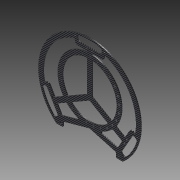
# Autodesk Inventor part: Bottom Plate
Saved by Autodesk Inventor 2015 (Build 190159000, 159)
## iProperties
Created: 2016-08-08
Part Number: Bottom Plate
Material: Generic
Document SubType Name: Modeling
Designer: James Yelland
Density: 1 g/cm^3
Appearance: Default
Mass: 31.8774 g
Surface Area: 332.808 cm^2
Volume: 31.8774 cm^3
Author: James Yelland
Autodesk Inventor part; units mm, degrees
ref_plane "YZ Plane" through (0, 0, 0) normal (1, 0, 0) x (0, 1, 0)
ref_plane "XZ Plane" through (0, 0, 0) normal (0, 1, 0) x (-1, 0, 0)
ref_plane "XY Plane" through (0, 0, 0) normal (0, 0, 1) x (1, 0, 0)
sketch "Sketch1" plane through (0, 0, 0) normal (0, 1, 0) x (-1, 0, 0)
  line L0 (-76.2102, -44) -> (-65.7102, -62.1865)
  line L1 (-67.1743, -67.6506) -> (-69.6351, -69.0713)
  line L2 (-94.6351, -25.7701) -> (-92.1743, -24.3494)
  line L3 (-86.7102, -25.8135) -> (-76.2102, -44)
  arc A0 (-96.4496, -30.438) -> (-74.5849, -68.3088) centre (0, 0) ccw
  arc A1 (-94.6351, -25.7701) -> (-96.4496, -30.438) centre (-92.6351, -29.2342) ccw
  arc A2 (-86.7102, -25.8135) -> (-92.1743, -24.3494) centre (-90.1743, -27.8135) ccw
  arc A3 (-67.1743, -67.6506) -> (-65.7102, -62.1865) centre (-69.1743, -64.1865) ccw
  arc A4 (-74.5849, -68.3088) -> (-69.6351, -69.0713) centre (-71.6351, -65.6072) ccw
  line L4 (76.2102, -44) -> (86.7102, -25.8135)
  line L5 (92.1743, -24.3494) -> (94.6351, -25.7701)
  line L6 (69.6351, -69.0713) -> (67.1743, -67.6506)
  line L7 (65.7102, -62.1865) -> (76.2102, -44)
  arc A5 (74.5849, -68.3088) -> (96.4496, -30.438) centre (0, 0) ccw
  arc A6 (69.6351, -69.0713) -> (74.5849, -68.3088) centre (71.6351, -65.6072) ccw
  arc A7 (65.7102, -62.1865) -> (67.1743, -67.6506) centre (69.1743, -64.1865) ccw
  arc A8 (92.1743, -24.3494) -> (86.7102, -25.8135) centre (90.1743, -27.8135) ccw
  arc A9 (96.4496, -30.438) -> (94.6351, -25.7701) centre (92.6351, -29.2342) ccw
  line L8 (0, 88) -> (-21, 88)
  line L9 (-25, 92) -> (-25, 94.8414)
  line L10 (25, 94.8414) -> (25, 92)
  line L11 (21, 88) -> (0, 88)
  arc A10 (21.8647, 98.7468) -> (-21.8647, 98.7468) centre (0, 0) ccw
  arc A11 (25, 94.8414) -> (21.8647, 98.7468) centre (21, 94.8414) ccw
  arc A12 (21, 88) -> (25, 92) centre (21, 92) ccw
  arc A13 (-25, 92) -> (-21, 88) centre (-21, 92) ccw
  arc A14 (-21.8647, 98.7468) -> (-25, 94.8414) centre (-21, 94.8414) ccw
  line L12 (-75.1122, -39.9019) -> (-77.6122, -35.5718)
  line L13 (-77.6122, -35.5718) -> (-75.8801, -34.5718)
  line L14 (-75.8801, -34.5718) -> (-73.3801, -38.9019)
  line L15 (-73.3801, -38.9019) -> (-75.1122, -39.9019)
  line L16 (-72.1122, -45.0981) -> (-69.6122, -49.4282)
  line L17 (-69.6122, -49.4282) -> (-67.8801, -48.4282)
  line L18 (-67.8801, -48.4282) -> (-70.3801, -44.0981)
  line L19 (-70.3801, -44.0981) -> (-72.1122, -45.0981)
  line L20 (72.1122, -45.0981) -> (69.6122, -49.4282)
  line L21 (69.6122, -49.4282) -> (67.8801, -48.4282)
  line L22 (67.8801, -48.4282) -> (70.3801, -44.0981)
  line L23 (70.3801, -44.0981) -> (72.1122, -45.0981)
  line L24 (73.3801, -38.9019) -> (75.1122, -39.9019)
  line L25 (75.8801, -34.5718) -> (73.3801, -38.9019)
  line L26 (77.6122, -35.5718) -> (75.8801, -34.5718)
  line L27 (75.1122, -39.9019) -> (77.6122, -35.5718)
  line L28 (3, 85) -> (8, 85)
  line L29 (8, 85) -> (8, 83)
  line L30 (8, 83) -> (3, 83)
  line L31 (3, 83) -> (3, 85)
  line L32 (-3, 83) -> (-3, 85)
  line L33 (-8, 83) -> (-3, 83)
  line L34 (-8, 85) -> (-8, 83)
  line L35 (-3, 85) -> (-8, 85)
  line L36 (0, 73.3) -> (-1.5, 73.3)
  line L37 (0, 73.3) -> (1.5, 73.3)
  line L38 (1.5, 73.3) -> (1.5, 74.8)
  line L39 (1.5, 74.8) -> (-1.5, 74.8)
  line L40 (-1.5, 74.8) -> (-1.5, 73.3)
  line L41 (0, 72.7) -> (-1.5, 72.7)
  line L42 (-1.5, 72.7) -> (-1.5, 71.2)
  line L43 (-1.5, 71.2) -> (1.5, 71.2)
  line L44 (1.5, 71.2) -> (1.5, 72.7)
  line L45 (1.5, 72.7) -> (0, 72.7)
  line L46 (-15.0457, 71.3993) -> (-16.5457, 71.3993)
  line L47 (-15.0457, 71.3993) -> (-13.5457, 71.3993)
  line L48 (-13.5457, 71.3993) -> (-13.5457, 72.8993)
  line L49 (-13.5457, 72.8993) -> (-16.5457, 72.8993)
  line L50 (-16.5457, 72.8993) -> (-16.5457, 71.3993)
  line L51 (-15.0457, 70.7993) -> (-16.5457, 70.7993)
  line L52 (-16.5457, 70.7993) -> (-16.5457, 69.2993)
  line L53 (-16.5457, 69.2993) -> (-13.5457, 69.2993)
  line L54 (-13.5457, 69.2993) -> (-13.5457, 70.7993)
  line L55 (-13.5457, 70.7993) -> (-15.0457, 70.7993)
  line L56 (-29.1461, 65.8166) -> (-30.6461, 65.8166)
  line L57 (-29.1461, 65.8166) -> (-27.6461, 65.8166)
  line L58 (-27.6461, 65.8166) -> (-27.6461, 67.3166)
  line L59 (-27.6461, 67.3166) -> (-30.6461, 67.3166)
  line L60 (-30.6461, 67.3166) -> (-30.6461, 65.8166)
  line L61 (-29.1461, 65.2166) -> (-30.6461, 65.2166)
  line L62 (-30.6461, 65.2166) -> (-30.6461, 63.7166)
  line L63 (-30.6461, 63.7166) -> (-27.6461, 63.7166)
  line L64 (-27.6461, 63.7166) -> (-27.6461, 65.2166)
  line L65 (-27.6461, 65.2166) -> (-29.1461, 65.2166)
  line L66 (-41.4151, 56.9026) -> (-42.9151, 56.9026)
  line L67 (-41.4151, 56.9026) -> (-39.9151, 56.9026)
  line L68 (-39.9151, 56.9026) -> (-39.9151, 58.4026)
  line L69 (-39.9151, 58.4026) -> (-42.9151, 58.4026)
  line L70 (-42.9151, 58.4026) -> (-42.9151, 56.9026)
  line L71 (-41.4151, 56.3026) -> (-42.9151, 56.3026)
  line L72 (-42.9151, 56.3026) -> (-42.9151, 54.8026)
  line L73 (-42.9151, 54.8026) -> (-39.9151, 54.8026)
  line L74 (-39.9151, 54.8026) -> (-39.9151, 56.3026)
  line L75 (-39.9151, 56.3026) -> (-41.4151, 56.3026)
  line L76 (-51.0818, 45.2175) -> (-52.5818, 45.2175)
  line L77 (-51.0818, 45.2175) -> (-49.5818, 45.2175)
  line L78 (-49.5818, 45.2175) -> (-49.5818, 46.7175)
  line L79 (-49.5818, 46.7175) -> (-52.5818, 46.7175)
  line L80 (-52.5818, 46.7175) -> (-52.5818, 45.2175)
  line L81 (-51.0818, 44.6175) -> (-52.5818, 44.6175)
  line L82 (-52.5818, 44.6175) -> (-52.5818, 43.1175)
  line L83 (-52.5818, 43.1175) -> (-49.5818, 43.1175)
  line L84 (-49.5818, 43.1175) -> (-49.5818, 44.6175)
  line L85 (-49.5818, 44.6175) -> (-51.0818, 44.6175)
  line L86 (-57.5389, 31.4955) -> (-59.0389, 31.4955)
  line L87 (-57.5389, 31.4955) -> (-56.0389, 31.4955)
  line L88 (-56.0389, 31.4955) -> (-56.0389, 32.9955)
  line L89 (-56.0389, 32.9955) -> (-59.0389, 32.9955)
  line L90 (-59.0389, 32.9955) -> (-59.0389, 31.4955)
  line L91 (-57.5389, 30.8955) -> (-59.0389, 30.8955)
  line L92 (-59.0389, 30.8955) -> (-59.0389, 29.3955)
  line L93 (-59.0389, 29.3955) -> (-56.0389, 29.3955)
  line L94 (-56.0389, 29.3955) -> (-56.0389, 30.8955)
  line L95 (-56.0389, 30.8955) -> (-57.5389, 30.8955)
  line L96 (-60.3806, 16.5988) -> (-61.8806, 16.5988)
  line L97 (-60.3806, 16.5988) -> (-58.8806, 16.5988)
  line L98 (-58.8806, 16.5988) -> (-58.8806, 18.0988)
  line L99 (-58.8806, 18.0988) -> (-61.8806, 18.0988)
  line L100 (-61.8806, 18.0988) -> (-61.8806, 16.5988)
  line L101 (-60.3806, 15.9988) -> (-61.8806, 15.9988)
  line L102 (-61.8806, 15.9988) -> (-61.8806, 14.4988)
  line L103 (-61.8806, 14.4988) -> (-58.8806, 14.4988)
  line L104 (-58.8806, 14.4988) -> (-58.8806, 15.9988)
  line L105 (-58.8806, 15.9988) -> (-60.3806, 15.9988)
  line L106 (-59.4284, 1.4634) -> (-60.9284, 1.4634)
  line L107 (-59.4284, 1.4634) -> (-57.9284, 1.4634)
  line L108 (-57.9284, 1.4634) -> (-57.9284, 2.9634)
  line L109 (-57.9284, 2.9634) -> (-60.9284, 2.9634)
  line L110 (-60.9284, 2.9634) -> (-60.9284, 1.4634)
  line L111 (-59.4284, 0.8634) -> (-60.9284, 0.8634)
  line L112 (-60.9284, 0.8634) -> (-60.9284, -0.6366)
  line L113 (-60.9284, -0.6366) -> (-57.9284, -0.6366)
  line L114 (-57.9284, -0.6366) -> (-57.9284, 0.8634)
  line L115 (-57.9284, 0.8634) -> (-59.4284, 0.8634)
  line L116 (-54.742, -12.9596) -> (-56.242, -12.9596)
  line L117 (-54.742, -12.9596) -> (-53.242, -12.9596)
  line L118 (-53.242, -12.9596) -> (-53.242, -11.4596)
  line L119 (-53.242, -11.4596) -> (-56.242, -11.4596)
  line L120 (-56.242, -11.4596) -> (-56.242, -12.9596)
  line L121 (-54.742, -13.5596) -> (-56.242, -13.5596)
  line L122 (-56.242, -13.5596) -> (-56.242, -15.0596)
  line L123 (-56.242, -15.0596) -> (-53.242, -15.0596)
  line L124 (-53.242, -15.0596) -> (-53.242, -13.5596)
  line L125 (-53.242, -13.5596) -> (-54.742, -13.5596)
  line L126 (-46.6161, -25.7642) -> (-48.1161, -25.7642)
  line L127 (-46.6161, -25.7642) -> (-45.1161, -25.7642)
  line L128 (-45.1161, -25.7642) -> (-45.1161, -24.2642)
  line L129 (-45.1161, -24.2642) -> (-48.1161, -24.2642)
  line L130 (-48.1161, -24.2642) -> (-48.1161, -25.7642)
  line L131 (-46.6161, -26.3642) -> (-48.1161, -26.3642)
  line L132 (-48.1161, -26.3642) -> (-48.1161, -27.8642)
  line L133 (-48.1161, -27.8642) -> (-45.1161, -27.8642)
  line L134 (-45.1161, -27.8642) -> (-45.1161, -26.3642)
  line L135 (-45.1161, -26.3642) -> (-46.6161, -26.3642)
  line L136 (-35.561, -36.1455) -> (-37.061, -36.1455)
  line L137 (-35.561, -36.1455) -> (-34.061, -36.1455)
  line L138 (-34.061, -36.1455) -> (-34.061, -34.6455)
  line L139 (-34.061, -34.6455) -> (-37.061, -34.6455)
  line L140 (-37.061, -34.6455) -> (-37.061, -36.1455)
  line L141 (-35.561, -36.7455) -> (-37.061, -36.7455)
  line L142 (-37.061, -36.7455) -> (-37.061, -38.2455)
  line L143 (-37.061, -38.2455) -> (-34.061, -38.2455)
  line L144 (-34.061, -38.2455) -> (-34.061, -36.7455)
  line L145 (-34.061, -36.7455) -> (-35.561, -36.7455)
  line L146 (-22.2715, -43.4515) -> (-23.7715, -43.4515)
  line L147 (-22.2715, -43.4515) -> (-20.7715, -43.4515)
  line L148 (-20.7715, -43.4515) -> (-20.7715, -41.9515)
  line L149 (-20.7715, -41.9515) -> (-23.7715, -41.9515)
  line L150 (-23.7715, -41.9515) -> (-23.7715, -43.4515)
  line L151 (-22.2715, -44.0515) -> (-23.7715, -44.0515)
  line L152 (-23.7715, -44.0515) -> (-23.7715, -45.5515)
  line L153 (-23.7715, -45.5515) -> (-20.7715, -45.5515)
  line L154 (-20.7715, -45.5515) -> (-20.7715, -44.0515)
  line L155 (-20.7715, -44.0515) -> (-22.2715, -44.0515)
  line L156 (-7.5827, -47.2229) -> (-9.0827, -47.2229)
  line L157 (-7.5827, -47.2229) -> (-6.0827, -47.2229)
  line L158 (-6.0827, -47.2229) -> (-6.0827, -45.7229)
  line L159 (-6.0827, -45.7229) -> (-9.0827, -45.7229)
  line L160 (-9.0827, -45.7229) -> (-9.0827, -47.2229)
  line L161 (-7.5827, -47.8229) -> (-9.0827, -47.8229)
  line L162 (-9.0827, -47.8229) -> (-9.0827, -49.3229)
  line L163 (-9.0827, -49.3229) -> (-6.0827, -49.3229)
  line L164 (-6.0827, -49.3229) -> (-6.0827, -47.8229)
  line L165 (-6.0827, -47.8229) -> (-7.5827, -47.8229)
  line L166 (7.5827, -47.2229) -> (6.0827, -47.2229)
  line L167 (7.5827, -47.2229) -> (9.0827, -47.2229)
  line L168 (9.0827, -47.2229) -> (9.0827, -45.7229)
  line L169 (9.0827, -45.7229) -> (6.0827, -45.7229)
  line L170 (6.0827, -45.7229) -> (6.0827, -47.2229)
  line L171 (7.5827, -47.8229) -> (6.0827, -47.8229)
  line L172 (6.0827, -47.8229) -> (6.0827, -49.3229)
  line L173 (6.0827, -49.3229) -> (9.0827, -49.3229)
  line L174 (9.0827, -49.3229) -> (9.0827, -47.8229)
  line L175 (9.0827, -47.8229) -> (7.5827, -47.8229)
  line L176 (22.2715, -43.4515) -> (20.7715, -43.4515)
  line L177 (22.2715, -43.4515) -> (23.7715, -43.4515)
  line L178 (23.7715, -43.4515) -> (23.7715, -41.9515)
  line L179 (23.7715, -41.9515) -> (20.7715, -41.9515)
  line L180 (20.7715, -41.9515) -> (20.7715, -43.4515)
  line L181 (22.2715, -44.0515) -> (20.7715, -44.0515)
  line L182 (20.7715, -44.0515) -> (20.7715, -45.5515)
  line L183 (20.7715, -45.5515) -> (23.7715, -45.5515)
  line L184 (23.7715, -45.5515) -> (23.7715, -44.0515)
  line L185 (23.7715, -44.0515) -> (22.2715, -44.0515)
  line L186 (35.561, -36.1455) -> (34.061, -36.1455)
  line L187 (35.561, -36.1455) -> (37.061, -36.1455)
  line L188 (37.061, -36.1455) -> (37.061, -34.6455)
  line L189 (37.061, -34.6455) -> (34.061, -34.6455)
  line L190 (34.061, -34.6455) -> (34.061, -36.1455)
  line L191 (35.561, -36.7455) -> (34.061, -36.7455)
  line L192 (34.061, -36.7455) -> (34.061, -38.2455)
  line L193 (34.061, -38.2455) -> (37.061, -38.2455)
  line L194 (37.061, -38.2455) -> (37.061, -36.7455)
  line L195 (37.061, -36.7455) -> (35.561, -36.7455)
  line L196 (46.6161, -25.7642) -> (45.1161, -25.7642)
  line L197 (46.6161, -25.7642) -> (48.1161, -25.7642)
  line L198 (48.1161, -25.7642) -> (48.1161, -24.2642)
  line L199 (48.1161, -24.2642) -> (45.1161, -24.2642)
  line L200 (45.1161, -24.2642) -> (45.1161, -25.7642)
  line L201 (46.6161, -26.3642) -> (45.1161, -26.3642)
  line L202 (45.1161, -26.3642) -> (45.1161, -27.8642)
  line L203 (45.1161, -27.8642) -> (48.1161, -27.8642)
  line L204 (48.1161, -27.8642) -> (48.1161, -26.3642)
  line L205 (48.1161, -26.3642) -> (46.6161, -26.3642)
  line L206 (54.742, -12.9596) -> (53.242, -12.9596)
  line L207 (54.742, -12.9596) -> (56.242, -12.9596)
  line L208 (56.242, -12.9596) -> (56.242, -11.4596)
  line L209 (56.242, -11.4596) -> (53.242, -11.4596)
  line L210 (53.242, -11.4596) -> (53.242, -12.9596)
  line L211 (54.742, -13.5596) -> (53.242, -13.5596)
  line L212 (53.242, -13.5596) -> (53.242, -15.0596)
  line L213 (53.242, -15.0596) -> (56.242, -15.0596)
  line L214 (56.242, -15.0596) -> (56.242, -13.5596)
  line L215 (56.242, -13.5596) -> (54.742, -13.5596)
  line L216 (59.4284, 1.4634) -> (57.9284, 1.4634)
  line L217 (59.4284, 1.4634) -> (60.9284, 1.4634)
  line L218 (60.9284, 1.4634) -> (60.9284, 2.9634)
  line L219 (60.9284, 2.9634) -> (57.9284, 2.9634)
  line L220 (57.9284, 2.9634) -> (57.9284, 1.4634)
  line L221 (59.4284, 0.8634) -> (57.9284, 0.8634)
  line L222 (57.9284, 0.8634) -> (57.9284, -0.6366)
  line L223 (57.9284, -0.6366) -> (60.9284, -0.6366)
  line L224 (60.9284, -0.6366) -> (60.9284, 0.8634)
  line L225 (60.9284, 0.8634) -> (59.4284, 0.8634)
  line L226 (60.3806, 16.5988) -> (58.8806, 16.5988)
  line L227 (60.3806, 16.5988) -> (61.8806, 16.5988)
  line L228 (61.8806, 16.5988) -> (61.8806, 18.0988)
  line L229 (61.8806, 18.0988) -> (58.8806, 18.0988)
  line L230 (58.8806, 18.0988) -> (58.8806, 16.5988)
  line L231 (60.3806, 15.9988) -> (58.8806, 15.9988)
  line L232 (58.8806, 15.9988) -> (58.8806, 14.4988)
  line L233 (58.8806, 14.4988) -> (61.8806, 14.4988)
  line L234 (61.8806, 14.4988) -> (61.8806, 15.9988)
  line L235 (61.8806, 15.9988) -> (60.3806, 15.9988)
  line L236 (57.5389, 31.4955) -> (56.0389, 31.4955)
  line L237 (57.5389, 31.4955) -> (59.0389, 31.4955)
  line L238 (59.0389, 31.4955) -> (59.0389, 32.9955)
  line L239 (59.0389, 32.9955) -> (56.0389, 32.9955)
  line L240 (56.0389, 32.9955) -> (56.0389, 31.4955)
  line L241 (57.5389, 30.8955) -> (56.0389, 30.8955)
  line L242 (56.0389, 30.8955) -> (56.0389, 29.3955)
  line L243 (56.0389, 29.3955) -> (59.0389, 29.3955)
  line L244 (59.0389, 29.3955) -> (59.0389, 30.8955)
  line L245 (59.0389, 30.8955) -> (57.5389, 30.8955)
  line L246 (51.0818, 45.2175) -> (49.5818, 45.2175)
  line L247 (51.0818, 45.2175) -> (52.5818, 45.2175)
  line L248 (52.5818, 45.2175) -> (52.5818, 46.7175)
  line L249 (52.5818, 46.7175) -> (49.5818, 46.7175)
  line L250 (49.5818, 46.7175) -> (49.5818, 45.2175)
  line L251 (51.0818, 44.6175) -> (49.5818, 44.6175)
  line L252 (49.5818, 44.6175) -> (49.5818, 43.1175)
  line L253 (49.5818, 43.1175) -> (52.5818, 43.1175)
  line L254 (52.5818, 43.1175) -> (52.5818, 44.6175)
  line L255 (52.5818, 44.6175) -> (51.0818, 44.6175)
  line L256 (41.4151, 56.9026) -> (39.9151, 56.9026)
  line L257 (41.4151, 56.9026) -> (42.9151, 56.9026)
  line L258 (42.9151, 56.9026) -> (42.9151, 58.4026)
  line L259 (42.9151, 58.4026) -> (39.9151, 58.4026)
  line L260 (39.9151, 58.4026) -> (39.9151, 56.9026)
  line L261 (41.4151, 56.3026) -> (39.9151, 56.3026)
  line L262 (39.9151, 56.3026) -> (39.9151, 54.8026)
  line L263 (39.9151, 54.8026) -> (42.9151, 54.8026)
  line L264 (42.9151, 54.8026) -> (42.9151, 56.3026)
  line L265 (42.9151, 56.3026) -> (41.4151, 56.3026)
  line L266 (29.1461, 65.8166) -> (27.6461, 65.8166)
  line L267 (29.1461, 65.8166) -> (30.6461, 65.8166)
  line L268 (30.6461, 65.8166) -> (30.6461, 67.3166)
  line L269 (30.6461, 67.3166) -> (27.6461, 67.3166)
  line L270 (27.6461, 67.3166) -> (27.6461, 65.8166)
  line L271 (29.1461, 65.2166) -> (27.6461, 65.2166)
  line L272 (27.6461, 65.2166) -> (27.6461, 63.7166)
  line L273 (27.6461, 63.7166) -> (30.6461, 63.7166)
  line L274 (30.6461, 63.7166) -> (30.6461, 65.2166)
  line L275 (30.6461, 65.2166) -> (29.1461, 65.2166)
  line L276 (15.0457, 71.3993) -> (13.5457, 71.3993)
  line L277 (15.0457, 71.3993) -> (16.5457, 71.3993)
  line L278 (16.5457, 71.3993) -> (16.5457, 72.8993)
  line L279 (16.5457, 72.8993) -> (13.5457, 72.8993)
  line L280 (13.5457, 72.8993) -> (13.5457, 71.3993)
  line L281 (15.0457, 70.7993) -> (13.5457, 70.7993)
  line L282 (13.5457, 70.7993) -> (13.5457, 69.2993)
  line L283 (13.5457, 69.2993) -> (16.5457, 69.2993)
  line L284 (16.5457, 69.2993) -> (16.5457, 70.7993)
  line L285 (16.5457, 70.7993) -> (15.0457, 70.7993)
  line L286 (54.0074, -78) -> (54.0074, -71.5202)
  line L287 (52.5426, -69.5932) -> (0.5352, -55.1487)
  line L288 (-54.0074, -78) -> (-54.0074, -71.5202)
  line L289 (-52.5426, -69.5932) -> (-0.5352, -55.1487)
  arc A15 (68.5743, -79.5146) -> (-68.5743, -79.5146) centre (0, 0) ccw
  line L290 (67.2681, -80) -> (56.0074, -80)
  line L291 (-56.0074, -80) -> (-67.2681, -80)
  arc A16 (54.0074, -78) -> (56.0074, -80) centre (56.0074, -78) ccw
  arc A17 (67.2681, -80) -> (68.5743, -79.5146) centre (67.2681, -78) ccw
  arc A18 (54.0074, -71.5202) -> (52.5426, -69.5932) centre (52.0074, -71.5202) ccw
  arc A19 (0.5352, -55.1487) -> (-0.5352, -55.1487) centre (0, -57.0757) ccw
  arc A20 (-52.5426, -69.5932) -> (-54.0074, -71.5202) centre (-52.0074, -71.5202) ccw
  arc A21 (-56.0074, -80) -> (-54.0074, -78) centre (-56.0074, -78) ccw
  arc A22 (-68.5743, -79.5146) -> (-67.2681, -80) centre (-67.2681, -78) ccw
  line L292 (-30, 85) -> (-30, 87.3212)
  line L293 (30, 85) -> (30, 87.3212)
  arc A23 (-30, 85) -> (-25, 80) centre (-25, 85) ccw
  arc A24 (25, 80) -> (30, 85) centre (25, 85) ccw
  circle A25 centre (-30, 95.3939) radius 1.6
  circle A26 centre (30, 95.3939) radius 1.6
  line L294 (-88.6122, -16.5192) -> (-90.6224, -17.6799)
  arc A27 (-81.782, -18.3494) -> (-88.6122, -16.5192) centre (-86.1122, -20.8494) ccw
  circle A28 centre (-59.2474, -74.7601) radius 1.6
  circle A29 centre (-97.6136, -21.7162) radius 1.6
  line L295 (88.6122, -16.5192) -> (90.6224, -17.6799)
  arc A30 (88.6122, -16.5192) -> (81.782, -18.3494) centre (86.1122, -20.8494) ccw
  circle A31 centre (97.6136, -21.7162) radius 1.6
  circle A32 centre (59.2474, -74.7601) radius 1.6
  arc A33 (-32.6882, 89.1991) -> (-93.5928, -16.2908) centre (0, 0) ccw
  arc A34 (93.5928, -16.2908) -> (32.6882, 89.1991) centre (0, 0) ccw
  arc A35 (-30, 87.3212) -> (-32.6882, 89.1991) centre (-32, 87.3212) ccw
  arc A36 (32.6882, 89.1991) -> (30, 87.3212) centre (32, 87.3212) ccw
  arc A37 (90.6224, -17.6799) -> (93.5928, -16.2908) centre (91.6224, -15.9478) ccw
  arc A38 (-93.5928, -16.2908) -> (-90.6224, -17.6799) centre (-91.6224, -15.9478) ccw
  line L296 (-55.7273, -60.4776) -> (-24.9522, -51.9302)
  line L297 (55.7273, -60.4776) -> (24.9522, -51.9302)
  arc A39 (-57.9945, -59.5505) -> (-55.7273, -60.4776) centre (-56.2625, -58.5505) ccw
  arc A40 (55.7273, -60.4776) -> (57.9945, -59.5505) centre (56.2625, -58.5505) ccw
  line L298 (-65.05, -43.3301) -> (-48.4689, -33.757)
  line L299 (-70.05, -34.6699) -> (-55.4501, -26.2406)
  line L300 (-35.7724, -26.4267) -> (-1, -6.3509)
  line L301 (-43.3011, -19.2264) -> (-6, 2.3094)
  line L302 (1, -6.3509) -> (35.7724, -26.4267)
  line L303 (48.4689, -33.757) -> (65.05, -43.3301)
  line L304 (55.4501, -26.2406) -> (70.05, -34.6699)
  line L305 (5, 4.0415) -> (5, 65.5401)
  line L306 (-5, 4.0415) -> (-5, 65.5401)
  line L307 (-5, 78.7288) -> (-5, 79)
  line L308 (5, 78.7288) -> (5, 79)
  line L309 (6, 2.3094) -> (43.3011, -19.2264)
  arc A41 (-7.2617, 67.5229) -> (-45.9572, -18.6156) centre (0, 12.5) ccw
  arc A42 (45.9572, -18.6156) -> (7.2617, 67.5229) centre (0, 12.5) ccw
  arc A43 (-36.0723, -29.6787) -> (36.0723, -29.6787) centre (0, 12.5) ccw
  arc A44 (54.7775, -23.412) -> (5.9098, 77.7328) centre (0, 12.5) ccw
  arc A45 (-5.9098, 77.7328) -> (-54.7775, -23.412) centre (0, 12.5) ccw
  arc A46 (-46.0624, -34.0672) -> (-24.7322, -48.1512) centre (0, 12.5) ccw
  arc A47 (24.7322, -48.1512) -> (46.0624, -34.0672) centre (0, 12.5) ccw
  arc A48 (-6, 2.3094) -> (-5, 4.0415) centre (-7, 4.0415) ccw
  arc A49 (5, 4.0415) -> (6, 2.3094) centre (7, 4.0415) ccw
  arc A50 (1, -6.3509) -> (-1, -6.3509) centre (0, -8.0829) ccw
  arc A51 (-5, 65.5401) -> (-7.2617, 67.5229) centre (-7, 65.5401) ccw
  arc A52 (7.2617, 67.5229) -> (5, 65.5401) centre (7, 65.5401) ccw
  arc A53 (43.3011, -19.2264) -> (45.9572, -18.6156) centre (44.3011, -17.4944) ccw
  arc A54 (36.0723, -29.6787) -> (35.7724, -26.4267) centre (34.7724, -28.1587) ccw
  arc A55 (-35.7724, -26.4267) -> (-36.0723, -29.6787) centre (-34.7724, -28.1587) ccw
  arc A56 (-45.9572, -18.6156) -> (-43.3011, -19.2264) centre (-44.3011, -17.4944) ccw
  arc A57 (24.7322, -48.1512) -> (24.9522, -51.9302) centre (25.4874, -50.0031) ccw
  arc A58 (48.4689, -33.757) -> (46.0624, -34.0672) centre (47.4689, -35.4891) ccw
  arc A59 (-24.9522, -51.9302) -> (-24.7322, -48.1512) centre (-25.4874, -50.0031) ccw
  arc A60 (-46.0624, -34.0672) -> (-48.4689, -33.757) centre (-47.4689, -35.4891) ccw
  arc A61 (-55.4501, -26.2406) -> (-54.7775, -23.412) centre (-56.4501, -24.5086) ccw
  arc A62 (54.7775, -23.412) -> (55.4501, -26.2406) centre (56.4501, -24.5086) ccw
  line L310 (-81.782, -18.3494) -> (-72.782, -33.9378)
  line L311 (-65.782, -46.0622) -> (-57.9945, -59.5505)
  line L312 (57.9945, -59.5505) -> (65.782, -46.0622)
  line L313 (72.782, -33.9378) -> (81.782, -18.3494)
  line L314 (-25, 80) -> (-6, 80)
  line L315 (6, 80) -> (25, 80)
  arc A63 (-65.05, -43.3301) -> (-65.782, -46.0622) centre (-64.05, -45.0622) ccw
  arc A64 (-72.782, -33.9378) -> (-70.05, -34.6699) centre (-71.05, -32.9378) ccw
  arc A65 (65.782, -46.0622) -> (65.05, -43.3301) centre (64.05, -45.0622) ccw
  arc A66 (70.05, -34.6699) -> (72.782, -33.9378) centre (71.05, -32.9378) ccw
  arc A67 (-5.9098, 77.7328) -> (-5, 78.7288) centre (-6, 78.7288) ccw
  arc A68 (-5, 79) -> (-6, 80) centre (-6, 79) ccw
  arc A69 (5, 78.7288) -> (5.9098, 77.7328) centre (6, 78.7288) ccw
  arc A70 (6, 80) -> (5, 79) centre (6, 79) ccw
  point P0 (-63.7102, -65.6506)
  point P1 (-72.3705, -70.6506)
  point P2 (-97.3705, -27.3494)
  point P3 (88.7102, -22.3494)
  point P4 (97.3705, -27.3494)
  point P5 (-25, 88)
  point P6 (-25, 98)
  point P7 (68.0074, -80)
  point P8 (-68.0074, -80)
  point P9 (-30, 80)
  point P10 (-30, 90.1388)
  point P11 (30, 80)
  point P12 (30, 90.1388)
  point P13 (-84.282, -14.0192)
  point P14 (-93.0625, -19.0886)
  point P15 (84.282, -14.0192)
  point P16 (93.0625, -19.0886)
  point P17 (-18.8389, -50.2323)
  point P18 (18.8389, -50.2323)
  point P19 (71.782, -35.6699)
  point P20 (66.782, -44.3301)
  point P21 (-5, 80)
  point P22 (5, 80)
  point P23 (-66.782, -44.3301)
  point P24 (-71.782, -35.6699)
  point P25 (-47.1315, -32.9849)
  point P26 (-53.5872, -25.1651)
  point P27 (-38.1564, -27.8031)
  point P28 (-44.8863, -20.1416)
  point P29 (38.1564, -27.8031)
  point P30 (47.1315, -32.9849)
  point P31 (53.5872, -25.1651)
  point P32 (5, 67.7743)
  point P33 (-5, 67.7743)
  point P34 (-5, 77.8089)
  point P35 (5, 77.8089)
  point P36 (44.8863, -20.1416)
  point P37 (-44.8863, -20.1416)
  dimension "d65" = 360
  dimension "d311" = 360
  dimension "d298" = 2
  dimension "d303" = 2
  dimension "d313" = 2
  dimension "d314" = 2
  dimension "d315" = 1
  constraints: 632 end point, 154 point on circle, 71 centre point, 71 point on line, 56 tangent, 24 equal radius, 8 coincident, 4 collinear, 1 horizontal, 7 other
  measures "d298" radius of A35
  measures "d303" radius of A39
  measures "d313" radius of A48
  measures "d314" radius of A63
  measures "d315" radius of A67
extrude "Extrusion1" add sketch "Sketch1" along normal blind 2
body "Solid1"
